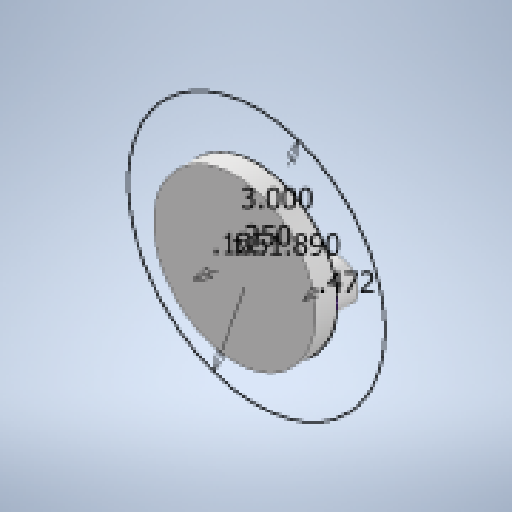
# Autodesk Inventor part: Temp - Gears
Saved by Autodesk Inventor 2023.2 (Build 272271000, 271)
## iProperties
Created: 2023-02-28
Part Number: Temp - Gears
Material: Generic
Document SubType Name: Modeling
Designer: Nathan Cai
Density: 1 g/cm^3
Appearance: Default
Author: Nathan Cai
Autodesk Inventor part; units mm, degrees
ref_plane "YZ Plane" through (0, 0, 0) normal (1, 0, 0) x (0, 1, 0)
ref_plane "XZ Plane" through (0, 0, 0) normal (0, 1, 0) x (-1, 0, 0)
ref_plane "XY Plane" through (0, 0, 0) normal (0, 0, 1) x (1, 0, 0)
sketch "Sketch1" plane through (0, 0, 0) normal (0, 0, 1) x (1, 0, 0)
  circle A0 centre (0, 0) radius 38.1
  circle A1 centre (0, 0) radius 24
  circle A2 centre (18, 0) radius 6
  line L0 (-24, 0) -> (24, 0) construction
  circle A3 centre (0, 0) radius 3.175
  circle A4 centre (0, 0) radius 6.35
  dimension "d2" = 12
  dimension "d0" = 76.2
  dimension "d1" = 48
  dimension "d3" = 6.35
  dimension "d4" = 3.175
  constraints: 4 centre point, 4 coincident, 2 end point, 2 point on circle, 1 horizontal alignment, 1 midpoint, 3 other
  measures "d0" diameter of A0
  measures "d1" diameter of A1
  measures "d3" diameter of A3
  measures "d4" radial gap between concentric circles of A3 A4
extrude "Extrusion1" add sketch "Sketch1" along normal blind 6.35 contours A1 | A2 | A4
extrude "Extrusion2" add sketch "Sketch1" against normal blind 6.35 contours A2
equation "\"d1\" = 4 * d2"
body "Solid1"
